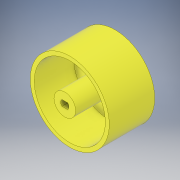
# Autodesk Inventor part: Wheel
Saved by Autodesk Inventor 2018 (Build 220112000, 112)
## iProperties
Created: 2018-01-12
Part Number: Wheel
Material: ABS Plastic
Document SubType Name: Modeling
Designer: Kyle
Density: 1.06 g/cm^3
Appearance: Smooth - Yellow
Author: Kyle
Autodesk Inventor part; units mm, degrees
ref_plane "YZ Plane" through (0, 0, 0) normal (1, 0, 0) x (0, 1, 0)
ref_plane "XZ Plane" through (0, 0, 0) normal (0, 1, 0) x (-1, 0, 0)
ref_plane "XY Plane" through (0, 0, 0) normal (0, 0, 1) x (1, 0, 0)
sketch "Sketch1" plane through (0, 0, 0) normal (0, 0, 1) x (1, 0, 0)
  circle A0 centre (0, 0) radius 25.4
  dimension "d0" = 50.8
  constraints: 1 centre point, 1 coincident
  measures "d0" diameter of A0
extrude "Extrusion1" add sketch "Sketch1" along normal blind 3.81
sketch "Sketch2" plane through (0, 0, 3.81) normal (0, 0, 1) x (1, 0, 0)
  circle A0 centre (0, 0) radius 22.86
  circle A1 centre (0, 0) radius 25.4
  dimension "d3" = 45.72
  constraints: 2 centre point, 2 coincident
  measures "d3" diameter of A0
extrude "Extrusion2" add sketch "Sketch2" along normal blind 25.4
sketch "Sketch3" plane through (0, 0, 3.81) normal (0, 0, 1) x (1, 0, 0)
  circle A0 centre (0, 0) radius 6.985
  dimension "d6" = 13.97
  constraints: 1 centre point, 1 coincident
  measures "d6" diameter of A0
extrude "Extrusion3" add sketch "Sketch3" along normal blind 28.575
sketch "Sketch4" plane through (0, 0, 32.385) normal (0, 0, 1) x (1, 0, 0)
  line L0 (-1.8665, 1.905) -> (1.8665, 1.905)
  line L1 (1.8665, -1.905) -> (-1.8665, -1.905)
  arc A0 (-1.8665, 1.905) -> (-1.8665, -1.905) centre (0, 0) ccw
  arc A1 (1.8665, -1.905) -> (1.8665, 1.905) centre (0, 0) ccw
  point P0 (0, 1.905)
  point P1 (0, -1.905)
  dimension "d10" = 1.905
  dimension "d11" = 1.905
  constraints: 4 end point, 4 point on circle, 2 centre point, 1 coincident, 1 horizontal, 1 parallel
  measures "d10" distance of point (0, 0) point (0, 1.905)
  measures "d11" distance of point (0, -1.905) point (0, 0)
extrude "Extrusion4" cut sketch "Sketch4" against normal blind 25.4
body "Solid1"
